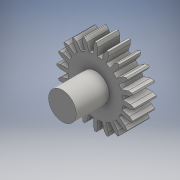
# Autodesk Inventor part: HelpGear
Saved by Autodesk Inventor 2016 SP1 (Build 200210100, 210)
## iProperties
Created: 2016-07-04
Part Number: HelpGear
Material: Generic
Document SubType Name: Modeling
Designer: Tore Den Store
Density: 1 g/cm^3
Appearance: Default
Author: Tore Den Store
Autodesk Inventor part; units mm, degrees
ref_plane "YZ Plane" through (0, 0, 0) normal (1, 0, 0) x (0, 1, 0)
ref_plane "XZ Plane" through (0, 0, 0) normal (0, 1, 0) x (-1, 0, 0)
ref_plane "XY Plane" through (0, 0, 0) normal (0, 0, 1) x (1, 0, 0)
sketch "Sketch1" plane through (0, 0, 0) normal (0, 1, 0) x (-1, 0, 0)
  circle A0 centre (0, 0) radius 25
  dimension "d0" = 50
  constraints: 1 centre point, 1 coincident
  measures "d0" diameter of A0
extrude "Extrusion1" add sketch "Sketch1" along normal blind 20
sketch "Sketch2" plane through (0, 0, 0) normal (0, -1, 0) x (1, 0, 0)
  circle A0 centre (0, 0) radius 25 projected
  line L0 (0, 0) -> (-1.9615, 24.9229)
  line L1 (0, 0) -> (1.9615, 24.9229)
  line L2 (0, 0) -> (40.2415, 0) construction
  line L3 (-1.9615, 24.9229) -> (-1.9615, 31.6715)
  line L4 (-1.9615, 31.6715) -> (-0.75, 35)
  line L5 (-0.75, 35) -> (0.75, 35)
  line L6 (0.75, 35) -> (1.9615, 31.6715)
  line L7 (1.9615, 31.6715) -> (1.9615, 24.9229)
  dimension "d3" = 9
  dimension "d4" = 85.5
  dimension "d5" = 10
  dimension "d6" = 110
  dimension "d7" = 110
  dimension "d8" = 1.5
  constraints: 16 end point, 2 parallel, 2 point on circle, 1 horizontal, 1 perpendicular, 1 vertical
  measures "d3" angle of L1 L0
  measures "d4" angle of L2 L1
  measures "d5" distance edge to line of A0 L5
  measures "d6" angle of L5 L4
  measures "d7" angle of L6 L5
  measures "d8" distance of L4.end L5.end
extrude "Extrusion2" add sketch "Sketch2" against normal blind 20 contours A0 L3 L4 L5 L6 L7
pattern_circular "Circular Pattern1" count 20 over 360 about axis through (0, 0, 0) along (0, 1, 0) of "Extrusion2"
sketch "Sketch3" plane through (0, 0, 0) normal (0, -1, 0) x (1, 0, 0)
  circle A0 centre (0, 0) radius 12.5
  dimension "d14" = 25
  constraints: 1 centre point, 1 coincident
  measures "d14" diameter of A0
extrude "Extrusion3" add sketch "Sketch3" along normal blind 30
equation "\"d7\" = d6"
body "Solid1"
